Autodesk Inventor part; units mm, degrees
(part 3 of 3)
  spline S427 degree 2 poles (356.5427, 51.4745) (356.6884, 51.4745) (356.9524, 51.4335) (357.0525, 51.4017) knots 0 0 0 1 2 2 2
  line L537 (357.0525, 51.4017) -> (358.4682, 51.4017)
  line L538 (358.4682, 51.4017) -> (358.4682, 50.8509)
  line L539 (358.4682, 50.8509) -> (357.8446, 50.8509)
  spline S428 degree 2 poles (355.7006, 50.1317) (355.7006, 49.945) (355.8235, 49.6309) (356.0511, 49.4125) (356.3561, 49.2941) (356.5472, 49.2941) knots 0 0 0 1 2 3 4 4 4
  spline S429 degree 2 poles (356.5472, 49.2941) (356.7475, 49.2941) (357.0616, 49.4307) (357.2756, 49.6628) (357.3894, 49.9678) (357.3894, 50.1317) knots 0 0 0 1 2 3 4 4 4
  spline S430 degree 2 poles (357.3894, 50.1317) (357.3894, 50.3137) (357.2665, 50.6278) (357.0389, 50.8463) (356.7339, 50.9647) (356.5472, 50.9647) knots 0 0 0 1 2 3 4 4 4
  spline S431 degree 2 poles (356.5472, 50.9647) (356.3424, 50.9647) (356.0283, 50.8236) (355.8144, 50.596) (355.7006, 50.291) (355.7006, 50.1317) knots 0 0 0 1 2 3 4 4 4
  spline S432 degree 2 poles (355.4957, 46.9362) (355.4957, 46.6631) (356.0693, 46.4081) (356.5837, 46.4081) knots 0 0 0 1 2 2 2
  spline S433 degree 2 poles (356.5837, 46.4081) (356.9068, 46.4081) (357.3438, 46.5265) (357.6124, 46.7131) (357.7308, 46.9589) (357.7308, 47.0864) knots 0 0 0 1 2 3 4 4 4
  spline S434 degree 2 poles (357.7308, 47.0864) (357.7308, 47.3231) (357.3438, 47.5507) (356.9433, 47.5689) knots 0 0 0 1 2 2 2
  line L540 (356.9433, 47.5689) -> (355.9236, 47.6053)
  spline S435 degree 2 poles (355.9236, 47.6053) (355.7962, 47.5188) (355.6277, 47.355) (355.5367, 47.1911) (355.4957, 47.0227) (355.4957, 46.9362) knots 0 0 0 1 2 3 4 4 4
  line L541 (360.7442, 50.8418) -> (359.588, 50.8418)
  line L542 (359.588, 50.8418) -> (359.588, 51.4017)
  line L543 (359.588, 51.4017) -> (361.427, 51.4017)
  line L544 (361.427, 51.4017) -> (361.427, 48.0651)
  line L545 (361.427, 48.0651) -> (362.5877, 48.0651)
  line L546 (362.5877, 48.0651) -> (362.5877, 47.5006)
  line L547 (362.5877, 47.5006) -> (359.4605, 47.5006)
  line L548 (359.4605, 47.5006) -> (359.4605, 48.0651)
  line L549 (359.4605, 48.0651) -> (360.7442, 48.0651)
  line L550 (360.7442, 48.0651) -> (360.7442, 50.8418)
  spline S436 degree 2 poles (360.9809, 53.0404) (361.0947, 53.0404) (361.2858, 52.9584) (361.4315, 52.8128) (361.5134, 52.6216) (361.5134, 52.5078) knots 0 0 0 1 2 3 4 4 4
  spline S437 degree 2 poles (361.5134, 52.5078) (361.5134, 52.3985) (361.4315, 52.2028) (361.2858, 52.0571) (361.0947, 51.9752) (360.9809, 51.9752) knots 0 0 0 1 2 3 4 4 4
  spline S438 degree 2 poles (360.9809, 51.9752) (360.8671, 51.9752) (360.6759, 52.0571) (360.5302, 52.2028) (360.4483, 52.3985) (360.4483, 52.5078) knots 0 0 0 1 2 3 4 4 4
  spline S439 degree 2 poles (360.4483, 52.5078) (360.4483, 52.6216) (360.5302, 52.8128) (360.6759, 52.9584) (360.8671, 53.0404) (360.9809, 53.0404) knots 0 0 0 1 2 3 4 4 4
  spline S440 degree 2 poles (366.9394, 47.5552) (366.7118, 47.4961) (366.2202, 47.446) (365.9653, 47.446) knots 0 0 0 1 2 2 2
  spline S441 degree 2 poles (365.9653, 47.446) (365.2324, 47.446) (364.5086, 48.1106) (364.5086, 48.7979) knots 0 0 0 1 2 2 2
  line L551 (364.5086, 48.7979) -> (364.5086, 50.8327)
  line L552 (364.5086, 50.8327) -> (363.4162, 50.8327)
  line L553 (363.4162, 50.8327) -> (363.4162, 51.4017)
  line L554 (363.4162, 51.4017) -> (364.5086, 51.4017)
  line L555 (364.5086, 51.4017) -> (364.5086, 52.4759)
  line L556 (364.5086, 52.4759) -> (365.1869, 52.6489)
  line L557 (365.1869, 52.6489) -> (365.1869, 51.4017)
  line L558 (365.1869, 51.4017) -> (366.9394, 51.4017)
  line L559 (366.9394, 51.4017) -> (366.9394, 50.8327)
  line L560 (366.9394, 50.8327) -> (365.1869, 50.8327)
  line L561 (365.1869, 50.8327) -> (365.1869, 48.8526)
  spline S442 degree 2 poles (365.1869, 48.8526) (365.1869, 48.4338) (365.633, 48.0195) (366.07, 48.0195) knots 0 0 0 1 2 2 2
  spline S443 degree 2 poles (366.07, 48.0195) (366.2566, 48.0195) (366.6981, 48.0787) (366.9394, 48.1379) knots 0 0 0 1 2 2 2
  line L562 (366.9394, 48.1379) -> (366.9394, 47.5552)
  line L563 (371.3138, 47.5006) -> (370.6356, 47.5006)
  line L564 (370.6356, 47.5006) -> (370.6356, 49.9951)
  spline S444 degree 2 poles (370.6356, 49.9951) (370.6356, 50.4457) (370.2987, 50.8918) (369.9847, 50.8918) knots 0 0 0 1 2 2 2
  spline S445 degree 2 poles (369.9847, 50.8918) (369.8481, 50.8918) (369.6114, 50.819) (369.3519, 50.6369) (369.0515, 50.3228) (368.8512, 50.0907) knots 0 0 0 1 2 3 4 4 4
  line L565 (368.8512, 50.0907) -> (368.8512, 47.5006)
  line L566 (368.8512, 47.5006) -> (368.173, 47.5006)
  line L567 (368.173, 47.5006) -> (368.173, 52.9949)
  line L568 (368.173, 52.9949) -> (368.8512, 52.9949)
  line L569 (368.8512, 52.9949) -> (368.8512, 51.4062)
  line L570 (368.8512, 51.4062) -> (368.8285, 50.7917)
  spline S446 degree 2 poles (368.8285, 50.7917) (368.9878, 50.9829) (369.2928, 51.2423) (369.6023, 51.4062) (369.9209, 51.4745) (370.0939, 51.4745) knots 0 0 0 1 2 3 4 4 4
  spline S447 degree 2 poles (370.0939, 51.4745) (370.6766, 51.4745) (371.3138, 50.7644) (371.3138, 50.0497) knots 0 0 0 1 2 2 2
  line L571 (371.3138, 50.0497) -> (371.3138, 47.5006)
  line L572 (375.6928, 47.5006) -> (375.0829, 47.5006)
  line L573 (375.0829, 47.5006) -> (375.0601, 48.1288)
  spline S448 degree 2 poles (375.0601, 48.1288) (374.8871, 47.9285) (374.573, 47.6599) (374.259, 47.4961) (373.9449, 47.4323) (373.7719, 47.4323) knots 0 0 0 1 2 3 4 4 4
  spline S449 degree 2 poles (373.7719, 47.4323) (373.1665, 47.4323) (372.552, 48.1379) (372.552, 48.8526) knots 0 0 0 1 2 2 2
  line L574 (372.552, 48.8526) -> (372.552, 51.4017)
  line L575 (372.552, 51.4017) -> (373.2302, 51.4017)
  line L576 (373.2302, 51.4017) -> (373.2302, 48.9072)
  spline S450 degree 2 poles (373.2302, 48.9072) (373.2302, 48.0104) (373.9085, 48.0104) knots 0 0 0 1 1 1
  spline S451 degree 2 poles (373.9085, 48.0104) (374.0314, 48.0104) (374.2681, 48.0833) (374.5275, 48.2654) (374.828, 48.5794) (375.0146, 48.8161) knots 0 0 0 1 2 3 4 4 4
  line L577 (375.0146, 48.8161) -> (375.0146, 51.4017)
  line L578 (375.0146, 51.4017) -> (375.6928, 51.4017)
  line L579 (375.6928, 51.4017) -> (375.6928, 47.5006)
  spline S452 degree 2 poles (380.2676, 49.5217) (380.2676, 49.0392) (379.999, 48.2699) (379.5074, 47.7373) (378.7973, 47.4551) (378.3557, 47.4551) knots 0 0 0 1 2 3 4 4 4
  spline S453 degree 2 poles (378.3557, 47.4551) (378.0098, 47.4551) (377.286, 47.5871) (376.931, 47.7328) knots 0 0 0 1 2 2 2
  line L580 (376.931, 47.7328) -> (376.931, 52.9949)
  line L581 (376.931, 52.9949) -> (377.6092, 52.9949)
  line L582 (377.6092, 52.9949) -> (377.6092, 51.4836)
  line L583 (377.6092, 51.4836) -> (377.5774, 50.7598)
  spline S454 degree 2 poles (377.5774, 50.7598) (377.8687, 51.1513) (378.5333, 51.4745) (378.9156, 51.4745) knots 0 0 0 1 2 2 2
  spline S455 degree 2 poles (378.9156, 51.4745) (379.2479, 51.4745) (379.7532, 51.1968) (380.0946, 50.687) (380.2676, 49.9678) (380.2676, 49.5217) knots 0 0 0 1 2 3 4 4 4
  spline S456 degree 2 poles (379.5757, 49.4898) (379.5757, 49.7994) (379.4846, 50.3092) (379.2934, 50.6779) (378.9885, 50.8827) (378.7791, 50.8827) knots 0 0 0 1 2 3 4 4 4
  spline S457 degree 2 poles (378.7791, 50.8827) (378.6516, 50.8827) (378.3876, 50.8008) (378.1008, 50.6096) (377.7867, 50.2955) (377.6092, 50.0634) knots 0 0 0 1 2 3 4 4 4
  line L584 (377.6092, 50.0634) -> (377.6092, 48.1698)
  spline S458 degree 2 poles (377.6092, 48.1698) (377.8095, 48.0924) (378.2192, 48.0013) (378.4058, 48.0013) knots 0 0 0 1 2 2 2
  spline S459 degree 2 poles (378.4058, 48.0013) (378.638, 48.0013) (379.0613, 48.147) (379.3845, 48.493) (379.5757, 49.0665) (379.5757, 49.4898) knots 0 0 0 1 2 3 4 4 4
  spline S460 degree 2 poles (382.844, 48.7251) (382.976, 48.7251) (383.2127, 48.625) (383.3902, 48.4474) (383.4904, 48.2107) (383.4904, 48.0742) knots 0 0 0 1 2 3 4 4 4
  spline S461 degree 2 poles (383.4904, 48.0742) (383.4904, 47.9422) (383.3902, 47.71) (383.2127, 47.5325) (382.976, 47.4323) (382.844, 47.4323) knots 0 0 0 1 2 3 4 4 4
  spline S462 degree 2 poles (382.844, 47.4323) (382.7074, 47.4323) (382.4753, 47.5325) (382.2977, 47.71) (382.1976, 47.9422) (382.1976, 48.0742) knots 0 0 0 1 2 3 4 4 4
  spline S463 degree 2 poles (382.1976, 48.0742) (382.1976, 48.2107) (382.2977, 48.4474) (382.4753, 48.625) (382.7074, 48.7251) (382.844, 48.7251) knots 0 0 0 1 2 3 4 4 4
  spline S464 degree 2 poles (388.7206, 47.6463) (388.4566, 47.5461) (387.9012, 47.446) (387.6053, 47.446) knots 0 0 0 1 2 2 2
  spline S465 degree 2 poles (387.6053, 47.446) (386.6813, 47.446) (385.6799, 48.4474) (385.6799, 49.4125) knots 0 0 0 1 2 2 2
  spline S466 degree 2 poles (385.6799, 49.4125) (385.6799, 49.8768) (385.9666, 50.6278) (386.4901, 51.165) (387.2139, 51.4563) (387.6463, 51.4563) knots 0 0 0 1 2 3 4 4 4
  spline S467 degree 2 poles (387.6463, 51.4563) (387.9513, 51.4563) (388.4793, 51.3698) (388.7206, 51.2742) knots 0 0 0 1 2 2 2
  line L585 (388.7206, 51.2742) -> (388.7206, 50.6278)
  spline S468 degree 2 poles (388.7206, 50.6278) (388.4657, 50.7598) (387.9422, 50.8827) (387.66, 50.8827) knots 0 0 0 1 2 2 2
  spline S469 degree 2 poles (387.66, 50.8827) (387.4005, 50.8827) (386.9362, 50.6825) (386.5857, 50.3092) (386.3854, 49.7721) (386.3854, 49.4352) knots 0 0 0 1 2 3 4 4 4
  spline S470 degree 2 poles (386.3854, 49.4352) (386.3854, 48.7297) (387.0728, 48.0241) (387.6873, 48.0241) knots 0 0 0 1 2 2 2
  spline S471 degree 2 poles (387.6873, 48.0241) (387.9604, 48.0241) (388.4793, 48.1516) (388.7206, 48.2745) knots 0 0 0 1 2 2 2
  line L586 (388.7206, 48.2745) -> (388.7206, 47.6463)
  spline S472 degree 2 poles (393.4637, 49.4853) (393.4637, 49.0301) (393.2088, 48.2699) (392.7263, 47.7328) (392.0344, 47.4323) (391.5929, 47.4323) knots 0 0 0 1 2 3 4 4 4
  spline S473 degree 2 poles (391.5929, 47.4323) (391.1741, 47.4323) (390.5095, 47.6918) (390.0498, 48.1971) (389.8039, 48.9436) (389.8039, 49.4307) knots 0 0 0 1 2 3 4 4 4
  spline S474 degree 2 poles (389.8039, 49.4307) (389.8039, 49.8859) (390.0589, 50.6369) (390.5414, 51.1741) (391.2333, 51.4745) (391.6748, 51.4745) knots 0 0 0 1 2 3 4 4 4
  spline S475 degree 2 poles (391.6748, 51.4745) (392.0936, 51.4745) (392.7582, 51.215) (393.2179, 50.7143) (393.4637, 49.9678) (393.4637, 49.4853) knots 0 0 0 1 2 3 4 4 4
  spline S476 degree 2 poles (392.7718, 49.4534) (392.7718, 49.8176) (392.6125, 50.3547) (392.3166, 50.7189) (391.8933, 50.9009) (391.6338, 50.9009) knots 0 0 0 1 2 3 4 4 4
  spline S477 degree 2 poles (391.6338, 50.9009) (391.3289, 50.9009) (390.901, 50.6642) (390.6233, 50.2682) (390.4958, 49.7447) (390.4958, 49.4534) knots 0 0 0 1 2 3 4 4 4
  spline S478 degree 2 poles (390.4958, 49.4534) (390.4958, 49.0938) (390.6552, 48.5521) (390.951, 48.188) (391.3698, 48.0059) (391.6338, 48.0059) knots 0 0 0 1 2 3 4 4 4
  spline S479 degree 2 poles (391.6338, 48.0059) (391.9388, 48.0059) (392.3667, 48.2426) (392.6444, 48.6386) (392.7718, 49.1621) (392.7718, 49.4534) knots 0 0 0 1 2 3 4 4 4
  line L587 (397.2328, 47.5006) -> (397.2328, 50.3046)
  spline S480 degree 2 poles (397.2328, 50.3046) (397.2328, 50.4867) (397.2055, 50.7189) (397.1508, 50.8554) (397.0689, 50.91) (397.0052, 50.91) knots 0 0 0 1 2 3 4 4 4
  spline S481 degree 2 poles (397.0052, 50.91) (396.9323, 50.91) (396.8094, 50.819) (396.6683, 50.6051) (396.4999, 50.2591) (396.3815, 50.0088) knots 0 0 0 1 2 3 4 4 4
  line L588 (396.3815, 50.0088) -> (396.3815, 47.5006)
  line L589 (396.3815, 47.5006) -> (395.7033, 47.5006)
  line L590 (395.7033, 47.5006) -> (395.7033, 50.2318)
  spline S482 degree 2 poles (395.7033, 50.2318) (395.7033, 50.4457) (395.676, 50.7098) (395.6214, 50.8554) (395.5349, 50.91) (395.4712, 50.91) knots 0 0 0 1 2 3 4 4 4
  spline S483 degree 2 poles (395.4712, 50.91) (395.4074, 50.91) (395.2891, 50.8327) (395.148, 50.6324) (394.9704, 50.2819) (394.8521, 50.0088) knots 0 0 0 1 2 3 4 4 4
  line L591 (394.8521, 50.0088) -> (394.8521, 47.5006)
  line L592 (394.8521, 47.5006) -> (394.1738, 47.5006)
  line L593 (394.1738, 47.5006) -> (394.1738, 51.4017)
  line L594 (394.1738, 51.4017) -> (394.7383, 51.4017)
  line L595 (394.7383, 51.4017) -> (394.7701, 50.6597)
  spline S484 degree 2 poles (394.7701, 50.6597) (394.8748, 50.8827) (395.066, 51.1923) (395.2663, 51.3835) (395.4985, 51.4745) (395.635, 51.4745) knots 0 0 0 1 2 3 4 4 4
  spline S485 degree 2 poles (395.635, 51.4745) (395.9537, 51.4745) (396.2814, 51.0603) (396.2814, 50.6278) knots 0 0 0 1 2 2 2
  spline S486 degree 2 poles (396.2814, 50.6278) (396.3724, 50.8327) (396.5545, 51.1468) (396.7594, 51.3607) (397.0097, 51.4745) (397.1736, 51.4745) knots 0 0 0 1 2 3 4 4 4
  spline S487 degree 2 poles (397.1736, 51.4745) (397.911, 51.4745) (397.911, 50.3411) knots 0 0 0 1 1 1
  line L596 (397.911, 50.3411) -> (397.911, 47.5006)
  line L597 (397.911, 47.5006) -> (397.2328, 47.5006)
  line L598 (401.9623, 52.9949) -> (399.2948, 46.6631)
  line L599 (399.2948, 46.6631) -> (398.6484, 46.6631)
  line L600 (398.6484, 46.6631) -> (401.3159, 52.9949)
  line L601 (401.3159, 52.9949) -> (401.9623, 52.9949)
  line L602 (406.7236, 47.5006) -> (405.8269, 47.5006)
  line L603 (405.8269, 47.5006) -> (404.7708, 48.9846)
  line L604 (404.7708, 48.9846) -> (403.7284, 47.5006)
  line L605 (403.7284, 47.5006) -> (402.8544, 47.5006)
  line L606 (402.8544, 47.5006) -> (404.3703, 49.458)
  line L607 (404.3703, 49.458) -> (402.9227, 51.4017)
  line L608 (402.9227, 51.4017) -> (403.7876, 51.4017)
  line L609 (403.7876, 51.4017) -> (404.8163, 49.8995)
  line L610 (404.8163, 49.8995) -> (405.8223, 51.4017)
  line L611 (405.8223, 51.4017) -> (406.6599, 51.4017)
  line L612 (406.6599, 51.4017) -> (405.1942, 49.4443)
  line L613 (405.1942, 49.4443) -> (406.7236, 47.5006)
  line L614 (410.3698, 47.5006) -> (410.3698, 50.3046)
  spline S488 degree 2 poles (410.3698, 50.3046) (410.3698, 50.4867) (410.3424, 50.7189) (410.2878, 50.8554) (410.2059, 50.91) (410.1422, 50.91) knots 0 0 0 1 2 3 4 4 4
  spline S489 degree 2 poles (410.1422, 50.91) (410.0693, 50.91) (409.9464, 50.819) (409.8053, 50.6051) (409.6369, 50.2591) (409.5185, 50.0088) knots 0 0 0 1 2 3 4 4 4
  line L615 (409.5185, 50.0088) -> (409.5185, 47.5006)
  line L616 (409.5185, 47.5006) -> (408.8403, 47.5006)
  line L617 (408.8403, 47.5006) -> (408.8403, 50.2318)
  spline S490 degree 2 poles (408.8403, 50.2318) (408.8403, 50.4457) (408.813, 50.7098) (408.7584, 50.8554) (408.6719, 50.91) (408.6081, 50.91) knots 0 0 0 1 2 3 4 4 4
  spline S491 degree 2 poles (408.6081, 50.91) (408.5444, 50.91) (408.4261, 50.8327) (408.2849, 50.6324) (408.1074, 50.2819) (407.9891, 50.0088) knots 0 0 0 1 2 3 4 4 4
  line L618 (407.9891, 50.0088) -> (407.9891, 47.5006)
  line L619 (407.9891, 47.5006) -> (407.3108, 47.5006)
  line L620 (407.3108, 47.5006) -> (407.3108, 51.4017)
  line L621 (407.3108, 51.4017) -> (407.8753, 51.4017)
  line L622 (407.8753, 51.4017) -> (407.9071, 50.6597)
  spline S492 degree 2 poles (407.9071, 50.6597) (408.0118, 50.8827) (408.203, 51.1923) (408.4033, 51.3835) (408.6355, 51.4745) (408.772, 51.4745) knots 0 0 0 1 2 3 4 4 4
  spline S493 degree 2 poles (408.772, 51.4745) (409.0906, 51.4745) (409.4184, 51.0603) (409.4184, 50.6278) knots 0 0 0 1 2 2 2
  spline S494 degree 2 poles (409.4184, 50.6278) (409.5094, 50.8327) (409.6915, 51.1468) (409.8963, 51.3607) (410.1467, 51.4745) (410.3106, 51.4745) knots 0 0 0 1 2 3 4 4 4
  spline S495 degree 2 poles (410.3106, 51.4745) (411.048, 51.4745) (411.048, 50.3411) knots 0 0 0 1 1 1
  line L623 (411.048, 50.3411) -> (411.048, 47.5006)
  line L624 (411.048, 47.5006) -> (410.3698, 47.5006)
  line L625 (415.1038, 47.5006) -> (414.4938, 47.5006)
  line L626 (414.4938, 47.5006) -> (414.4711, 48.1288)
  spline S496 degree 2 poles (414.4711, 48.1288) (414.2981, 47.9285) (413.984, 47.6599) (413.6699, 47.4961) (413.3558, 47.4323) (413.1829, 47.4323) knots 0 0 0 1 2 3 4 4 4
  spline S497 degree 2 poles (413.1829, 47.4323) (412.5775, 47.4323) (411.9629, 48.1379) (411.9629, 48.8526) knots 0 0 0 1 2 2 2
  line L627 (411.9629, 48.8526) -> (411.9629, 51.4017)
  line L628 (411.9629, 51.4017) -> (412.6412, 51.4017)
  line L629 (412.6412, 51.4017) -> (412.6412, 48.9072)
  spline S498 degree 2 poles (412.6412, 48.9072) (412.6412, 48.0104) (413.3194, 48.0104) knots 0 0 0 1 1 1
  spline S499 degree 2 poles (413.3194, 48.0104) (413.4423, 48.0104) (413.679, 48.0833) (413.9385, 48.2654) (414.2389, 48.5794) (414.4256, 48.8161) knots 0 0 0 1 2 3 4 4 4
  line L630 (414.4256, 48.8161) -> (414.4256, 51.4017)
  line L631 (414.4256, 51.4017) -> (415.1038, 51.4017)
  line L632 (415.1038, 51.4017) -> (415.1038, 47.5006)
  spline S500 degree 2 poles (419.4874, 47.5552) (419.2598, 47.4961) (418.7681, 47.446) (418.5132, 47.446) knots 0 0 0 1 2 2 2
  spline S501 degree 2 poles (418.5132, 47.446) (417.7804, 47.446) (417.0566, 48.1106) (417.0566, 48.7979) knots 0 0 0 1 2 2 2
  line L633 (417.0566, 48.7979) -> (417.0566, 50.8327)
  line L634 (417.0566, 50.8327) -> (415.9641, 50.8327)
  line L635 (415.9641, 50.8327) -> (415.9641, 51.4017)
  line L636 (415.9641, 51.4017) -> (417.0566, 51.4017)
  line L637 (417.0566, 51.4017) -> (417.0566, 52.4759)
  line L638 (417.0566, 52.4759) -> (417.7348, 52.6489)
  line L639 (417.7348, 52.6489) -> (417.7348, 51.4017)
  line L640 (417.7348, 51.4017) -> (419.4874, 51.4017)
  line L641 (419.4874, 51.4017) -> (419.4874, 50.8327)
  line L642 (419.4874, 50.8327) -> (417.7348, 50.8327)
  line L643 (417.7348, 50.8327) -> (417.7348, 48.8526)
  spline S502 degree 2 poles (417.7348, 48.8526) (417.7348, 48.4338) (418.1809, 48.0195) (418.6179, 48.0195) knots 0 0 0 1 2 2 2
  spline S503 degree 2 poles (418.6179, 48.0195) (418.8046, 48.0195) (419.2461, 48.0787) (419.4874, 48.1379) knots 0 0 0 1 2 2 2
  line L644 (419.4874, 48.1379) -> (419.4874, 47.5552)
  line L645 (423.2291, 47.5006) -> (423.2154, 48.0241)
  spline S504 degree 2 poles (423.2154, 48.0241) (422.8968, 47.71) (422.2367, 47.4323) (421.8771, 47.4323) knots 0 0 0 1 2 2 2
  spline S505 degree 2 poles (421.8771, 47.4323) (421.5403, 47.4323) (421.0669, 47.6053) (420.7619, 47.9012) (420.6162, 48.3063) (420.6162, 48.543) knots 0 0 0 1 2 3 4 4 4
  spline S506 degree 2 poles (420.6162, 48.543) (420.6162, 49.1302) (421.4902, 49.7948) (422.346, 49.7948) knots 0 0 0 1 2 2 2
  line L646 (422.346, 49.7948) -> (423.1562, 49.7948)
  line L647 (423.1562, 49.7948) -> (423.1562, 50.1362)
  spline S507 degree 2 poles (423.1562, 50.1362) (423.1562, 50.4822) (422.7147, 50.9009) (422.2595, 50.9009) knots 0 0 0 1 2 2 2
  spline S508 degree 2 poles (422.2595, 50.9009) (421.9272, 50.9009) (421.2854, 50.7553) (420.944, 50.6187) knots 0 0 0 1 2 2 2
  line L648 (420.944, 50.6187) -> (420.944, 51.2287)
  spline S509 degree 2 poles (420.944, 51.2287) (421.0714, 51.2742) (421.3855, 51.3652) (421.736, 51.4335) (422.1184, 51.4745) (422.3096, 51.4745) knots 0 0 0 1 2 3 4 4 4
  spline S510 degree 2 poles (422.3096, 51.4745) (422.6646, 51.4745) (423.2336, 51.3197) (423.6251, 51.0011) (423.8345, 50.5186) (423.8345, 50.1908) knots 0 0 0 1 2 3 4 4 4
  line L649 (423.8345, 50.1908) -> (423.8345, 47.5006)
  line L650 (423.8345, 47.5006) -> (423.2291, 47.5006)
  line L651 (423.1562, 49.2759) -> (422.2959, 49.2759)
  spline S511 degree 2 poles (422.2959, 49.2759) (422.041, 49.2759) (421.6768, 49.1757) (421.4447, 48.9891) (421.3309, 48.7297) (421.3309, 48.5658) knots 0 0 0 1 2 3 4 4 4
  spline S512 degree 2 poles (421.3309, 48.5658) (421.3309, 48.452) (421.3992, 48.2471) (421.5585, 48.0878) (421.8043, 47.9968) (421.9864, 47.9968) knots 0 0 0 1 2 3 4 4 4
  spline S513 degree 2 poles (421.9864, 47.9968) (422.2185, 47.9968) (422.8194, 48.279) (423.1562, 48.584) knots 0 0 0 1 2 2 2
  line L652 (423.1562, 48.584) -> (423.1562, 49.2759)
  line L653 (425.0999, 51.4017) -> (425.7053, 51.4017)
  line L654 (425.7053, 51.4017) -> (425.7327, 50.7735)
  spline S514 degree 2 poles (425.7327, 50.7735) (425.9011, 50.9738) (426.2197, 51.2423) (426.5293, 51.4062) (426.8479, 51.4745) (427.0209, 51.4745) knots 0 0 0 1 2 3 4 4 4
  spline S515 degree 2 poles (427.0209, 51.4745) (427.6217, 51.4745) (428.2408, 50.7644) (428.2408, 50.0497) knots 0 0 0 1 2 2 2
  line L655 (428.2408, 50.0497) -> (428.2408, 47.5006)
  line L656 (428.2408, 47.5006) -> (427.5625, 47.5006)
  line L657 (427.5625, 47.5006) -> (427.5625, 49.9951)
  spline S516 degree 2 poles (427.5625, 49.9951) (427.5625, 50.4503) (427.2212, 50.8918) (426.8843, 50.8918) knots 0 0 0 1 2 2 2
  spline S517 degree 2 poles (426.8843, 50.8918) (426.7569, 50.8918) (426.5201, 50.819) (426.2652, 50.6369) (425.9648, 50.3228) (425.7782, 50.0907) knots 0 0 0 1 2 3 4 4 4
  line L658 (425.7782, 50.0907) -> (425.7782, 47.5006)
  line L659 (425.7782, 47.5006) -> (425.0999, 47.5006)
  line L660 (425.0999, 47.5006) -> (425.0999, 51.4017)
  spline S518 degree 2 poles (432.6243, 47.5552) (432.3967, 47.4961) (431.9051, 47.446) (431.6502, 47.446) knots 0 0 0 1 2 2 2
  spline S519 degree 2 poles (431.6502, 47.446) (430.9174, 47.446) (430.1936, 48.1106) (430.1936, 48.7979) knots 0 0 0 1 2 2 2
  line L661 (430.1936, 48.7979) -> (430.1936, 50.8327)
  line L662 (430.1936, 50.8327) -> (429.1011, 50.8327)
  line L663 (429.1011, 50.8327) -> (429.1011, 51.4017)
  line L664 (429.1011, 51.4017) -> (430.1936, 51.4017)
  line L665 (430.1936, 51.4017) -> (430.1936, 52.4759)
  line L666 (430.1936, 52.4759) -> (430.8718, 52.6489)
  line L667 (430.8718, 52.6489) -> (430.8718, 51.4017)
  line L668 (430.8718, 51.4017) -> (432.6243, 51.4017)
  line L669 (432.6243, 51.4017) -> (432.6243, 50.8327)
  line L670 (432.6243, 50.8327) -> (430.8718, 50.8327)
  line L671 (430.8718, 50.8327) -> (430.8718, 48.8526)
  spline S520 degree 2 poles (430.8718, 48.8526) (430.8718, 48.4338) (431.3179, 48.0195) (431.7549, 48.0195) knots 0 0 0 1 2 2 2
  spline S521 degree 2 poles (431.7549, 48.0195) (431.9415, 48.0195) (432.3831, 48.0787) (432.6243, 48.1379) knots 0 0 0 1 2 2 2
  line L672 (432.6243, 48.1379) -> (432.6243, 47.5552)
  spline S522 degree 2 poles (436.9442, 48.5658) (436.9442, 48.3609) (436.8031, 48.0332) (436.5618, 47.7828) (436.2432, 47.6053) (435.8836, 47.487) (435.5012, 47.4323) (435.3191, 47.4323) knots 0 0 0 1 2 3 4 5 6 6 6
  spline S523 degree 2 poles (435.3191, 47.4323) (434.9231, 47.4323) (434.2585, 47.5052) (433.9399, 47.5826) knots 0 0 0 1 2 2 2
  line L673 (433.9399, 47.5826) -> (433.9399, 48.2062)
  spline S524 degree 2 poles (433.9399, 48.2062) (434.2813, 48.106) (434.9595, 48.0059) (435.2918, 48.0059) knots 0 0 0 1 2 2 2
  spline S525 degree 2 poles (435.2918, 48.0059) (435.7789, 48.0059) (436.2432, 48.2699) (436.2432, 48.5112) knots 0 0 0 1 2 2 2
  spline S526 degree 2 poles (436.2432, 48.5112) (436.2432, 48.6159) (436.1703, 48.7843) (435.9746, 48.9345) (435.5695, 49.0984) (435.2144, 49.2031) knots 0 0 0 1 2 3 4 4 4
  spline S527 degree 2 poles (435.2144, 49.2031) (434.9504, 49.2804) (434.5043, 49.4807) (434.1766, 49.7538) (433.9899, 50.118) (433.9899, 50.3684) knots 0 0 0 1 2 3 4 4 4
  spline S528 degree 2 poles (433.9899, 50.3684) (433.9899, 50.5322) (434.1401, 50.9192) (434.5089, 51.2514) (435.1279, 51.4745) (435.5968, 51.4745) knots 0 0 0 1 2 3 4 4 4
  spline S529 degree 2 poles (435.5968, 51.4745) (435.8244, 51.4745) (436.3843, 51.4244) (436.6893, 51.3607) knots 0 0 0 1 2 2 2
  line L674 (436.6893, 51.3607) -> (436.6893, 50.7598)
  spline S530 degree 2 poles (436.6893, 50.7598) (436.3706, 50.8372) (435.7971, 50.91) (435.5877, 50.91) knots 0 0 0 1 2 2 2
  spline S531 degree 2 poles (435.5877, 50.91) (435.3373, 50.91) (434.9914, 50.8327) (434.7774, 50.6961) (434.6818, 50.514) (434.6818, 50.4093) knots 0 0 0 1 2 3 4 4 4
  spline S532 degree 2 poles (434.6818, 50.4093) (434.6818, 50.3046) (434.7638, 50.1317) (434.9868, 49.9723) (435.3828, 49.813) (435.7015, 49.722) knots 0 0 0 1 2 3 4 4 4
  spline S533 degree 2 poles (435.7015, 49.722) (436.0474, 49.6218) (436.5208, 49.3988) (436.8167, 49.1257) (436.9442, 48.7843) (436.9442, 48.5658) knots 0 0 0 1 2 3 4 4 4
  spline S534 degree 2 poles (441.6327, 49.4853) (441.6327, 49.0301) (441.3778, 48.2699) (440.8953, 47.7328) (440.2034, 47.4323) (439.7618, 47.4323) knots 0 0 0 1 2 3 4 4 4
  spline S535 degree 2 poles (439.7618, 47.4323) (439.3431, 47.4323) (438.6785, 47.6918) (438.2187, 48.1971) (437.9729, 48.9436) (437.9729, 49.4307) knots 0 0 0 1 2 3 4 4 4
  spline S536 degree 2 poles (437.9729, 49.4307) (437.9729, 49.8859) (438.2278, 50.6369) (438.7103, 51.1741) (439.4022, 51.4745) (439.8438, 51.4745) knots 0 0 0 1 2 3 4 4 4
  spline S537 degree 2 poles (439.8438, 51.4745) (440.2625, 51.4745) (440.9271, 51.215) (441.3869, 50.7143) (441.6327, 49.9678) (441.6327, 49.4853) knots 0 0 0 1 2 3 4 4 4
  spline S538 degree 2 poles (440.9408, 49.4534) (440.9408, 49.8176) (440.7815, 50.3547) (440.4856, 50.7189) (440.0623, 50.9009) (439.8028, 50.9009) knots 0 0 0 1 2 3 4 4 4
  spline S539 degree 2 poles (439.8028, 50.9009) (439.4978, 50.9009) (439.0699, 50.6642) (438.7923, 50.2682) (438.6648, 49.7447) (438.6648, 49.4534) knots 0 0 0 1 2 3 4 4 4
  spline S540 degree 2 poles (438.6648, 49.4534) (438.6648, 49.0938) (438.8241, 48.5521) (439.12, 48.188) (439.5388, 48.0059) (439.8028, 48.0059) knots 0 0 0 1 2 3 4 4 4
  spline S541 degree 2 poles (439.8028, 48.0059) (440.1078, 48.0059) (440.5357, 48.2426) (440.8133, 48.6386) (440.9408, 49.1621) (440.9408, 49.4534) knots 0 0 0 1 2 3 4 4 4
  line L675 (442.6159, 51.4017) -> (443.2213, 51.4017)
  line L676 (443.2213, 51.4017) -> (443.2486, 50.7735)
  spline S542 degree 2 poles (443.2486, 50.7735) (443.4171, 50.9738) (443.7357, 51.2423) (444.0452, 51.4062) (444.3639, 51.4745) (444.5369, 51.4745) knots 0 0 0 1 2 3 4 4 4
  spline S543 degree 2 poles (444.5369, 51.4745) (445.1377, 51.4745) (445.7568, 50.7644) (445.7568, 50.0497) knots 0 0 0 1 2 2 2
  line L677 (445.7568, 50.0497) -> (445.7568, 47.5006)
  line L678 (445.7568, 47.5006) -> (445.0785, 47.5006)
  line L679 (445.0785, 47.5006) -> (445.0785, 49.9951)
  spline S544 degree 2 poles (445.0785, 49.9951) (445.0785, 50.4503) (444.7371, 50.8918) (444.4003, 50.8918) knots 0 0 0 1 2 2 2
  spline S545 degree 2 poles (444.4003, 50.8918) (444.2728, 50.8918) (444.0361, 50.819) (443.7812, 50.6369) (443.4808, 50.3228) (443.2942, 50.0907) knots 0 0 0 1 2 3 4 4 4
  line L680 (443.2942, 50.0907) -> (443.2942, 47.5006)
  line L681 (443.2942, 47.5006) -> (442.6159, 47.5006)
  line L682 (442.6159, 47.5006) -> (442.6159, 51.4017)
  point P0 (0, 0)
  dimension "d45" = 31.75
  dimension "d46" = 95.25
  dimension "d47" = 101.6
  dimension "d48" = 50.8
  dimension "d49" = 34.925
  dimension "d50" = 45
  dimension "d51" = 17.9693
  dimension "d55" = 1.5875
  dimension "d56" = 1.5875
  dimension "d57" = 1.27
  dimension "d58" = 1.27
  dimension "d59" = 0
  constraints: 20 end point, 3 horizontal, 2 parallel, 2 perpendicular, 2 point on line, 1 midpoint, 4 other
  measures "d45" distance from line of L5 L0.start
  measures "d46" distance from line of L5 L0.end
  measures "d47" distance from line of L6 L0.start
  measures "d48" distance from line of L6 L0.end
  measures "d49" distance of L0.end L2.start
  measures "d50" angle of L1 L2
  measures "d51" distance of L2.end L3.end
  measures "d55" distance between parallel lines of L1 L15
  measures "d56" distance between parallel lines of L1 L17
  measures "d57" distance between parallel lines of L18 L0
  measures "d58" distance between parallel lines of L0 L16
  measures "d59" angle of L5 L19
extrude "Extrusion3" cut sketch "Sketch3" against normal blind 0.0254
body "Solid1"
